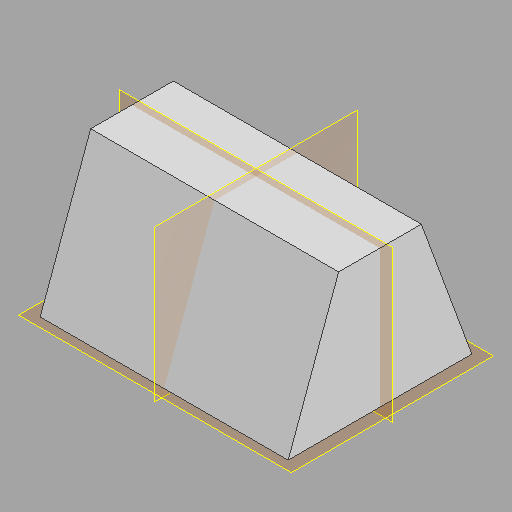
# Autodesk Inventor part: 9mm-STD-NIB
Saved by Autodesk Inventor 2025.4 (Build 294407000, 407)
## iProperties
Created: 2026-10-05
Part Number: 9mm-STD-NIB
Material: Generic
Document SubType Name: Modeling
Designer: phil.skelton
Density: 1 g/cm^3
Appearance: Default
Author: phil.skelton
Autodesk Inventor part; units mm, degrees
sketch "Sketch1" plane through (0, 0, 0) normal (1, 0, 0) x (0, 1, 0)
  line L0 (0, 2.6) -> (5, 2.6) construction
  line L1 (5, 2.6) -> (5, -2.6) construction
  line L2 (5, -2.6) -> (0, -2.6) construction
  line L3 (0, -2.6) -> (0, 2.6)
  line L4 (5, 1.5) -> (5, -1.5)
  line L5 (5, 1.5) -> (2, 2.6)
  line L6 (5, -1.5) -> (2, -2.6)
  line L7 (2, 2.6) -> (0, 2.6) construction
  line L8 (2, -2.6) -> (0, -2.6) construction
  line L9 (2, 2.6) -> (2, -2.6) construction
  line L10 (2, 2.6) -> (0, 3.3333)
  line L11 (0, 3.3333) -> (0, 2.6)
  line L12 (0, -2.6) -> (0, -3.3333)
  line L13 (0, -3.3333) -> (2, -2.6)
  point P0 (0, 0)
  point P1 (2.5, 2.6)
  point P2 (2.5, -2.6)
  point P3 (0, 0)
  dimension "d15" = 5.2
  dimension "d16" = 2.6
  dimension "d17" = 5
  dimension "d18" = 0
  dimension "d19" = 3
  dimension "d20" = 1.5
  dimension "d21" = 2
  constraints: 28 end point, 5 collinear, 5 point on line, 3 midpoint, 2 horizontal, 2 parallel, 1 perpendicular, 1 vertical, 1 vertical alignment
  measures "d15" distance of L8.end L3.end
  measures "d16" distance from line of point (0, 0) L0
  measures "d17" distance between parallel lines of L1 L3
  measures "d18" distance from line of point (0, 0) L3
  measures "d19" distance of L4.start L6.start
  measures "d20" vertical distance of point (0, 0) L4.start
  measures "d21" distance from line of L3 L7.start
extrude "Extrusion1" add sketch "Sketch1" along normal mid plane 9
equation "\"d16\" = 0.5 * d15"
equation "\"d20\" = 0.5 * d19"
body "Solid1"
